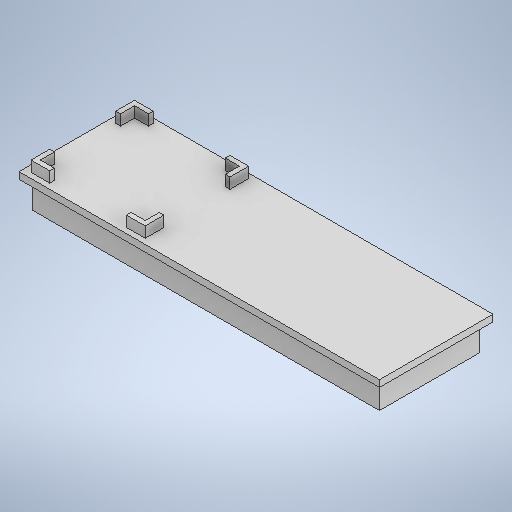
# Autodesk Inventor part: jugglingGloveCap
Saved by Autodesk Inventor 2025 (Build 290162010, 162A)
## iProperties
Created: 2024-07-10
Part Number: jugglingGloveCap
Material: Generic
Document SubType Name: Modeling
Designer: Dresden_Student
Density: 1 g/cm^3
Appearance: Default
Author: Dresden_Student
Autodesk Inventor part; units mm, degrees
ref_plane "YZ Plane" through (0, 0, 0) normal (1, 0, 0) x (0, 1, 0)
ref_plane "XZ Plane" through (0, 0, 0) normal (0, 1, 0) x (-1, 0, 0)
ref_plane "XY Plane" through (0, 0, 0) normal (0, 0, 1) x (1, 0, 0)
sketch "Sketch1" plane through (0, 0, 0) normal (0, 1, 0) x (-1, 0, 0)
  line L0 (-65, -18.75) -> (65, -18.75)
  line L1 (65, -18.75) -> (65, 18.75)
  line L2 (65, 18.75) -> (-65, 18.75)
  line L3 (-65, 18.75) -> (-65, -18.75)
  line L4 (-65, -18.75) -> (65, 18.75) construction
  line L5 (65, -18.75) -> (-65, 18.75) construction
  line L6 (61.5, 15.25) -> (-61.5, 15.25)
  line L7 (-61.5, 15.25) -> (-61.5, -15.25)
  line L8 (-61.5, -15.25) -> (61.5, -15.25)
  line L9 (61.5, -15.25) -> (61.5, 15.25)
  line L10 (61.5, 15.25) -> (-61.5, -15.25) construction
  line L11 (-61.5, 15.25) -> (61.5, -15.25) construction
  point P0 (0, 0)
  point P1 (0, 0)
  point P2 (61.5, 0)
  dimension "d0" = 37.5
  dimension "d1" = 130
  dimension "d2" = 3.5
  dimension "d3" = 3.5
  dimension "d4" = 3.5
  dimension "d5" = 3.5
  constraints: 24 end point, 5 midpoint, 4 parallel, 2 horizontal, 2 perpendicular
  measures "d0" distance of L0.end L1.end
  measures "d1" distance of L0.start L0.end
  measures "d2" distance from line of L1 point (61.5, 0)
  measures "d3" distance between parallel lines of L2 L6
  measures "d4" distance between parallel lines of L0 L8
  measures "d5" distance between parallel lines of L3 L7
extrude "Extrusion1" add sketch "Sketch1" against normal blind 2.5 contours L3 L2 L1 L0 | L9 L8 L7 L6
sketch "Sketch2" plane through (0, -2.5, 0) normal (0, -1, 0) x (1, 0, 0)
  point P0 (0, 0)
sketch "Sketch3" plane through (0, -2.5, 0) normal (0, -1, 0) x (1, 0, 0)
  line L0 (-63.875, -17.875) -> (63.875, -17.875)
  line L1 (63.875, -17.875) -> (63.875, 17.875)
  line L2 (63.875, 17.875) -> (-63.875, 17.875)
  line L3 (-63.875, 17.875) -> (-63.875, -17.875)
  line L4 (-63.875, -17.875) -> (63.875, 17.875) construction
  line L5 (63.875, -17.875) -> (-63.875, 17.875) construction
  line L6 (65, 18.75) -> (-65, 18.75) projected
  line L7 (65, -18.75) -> (65, 18.75) projected
  line L8 (-65, 18.75) -> (65, 18.75)
  line L9 (65, 18.75) -> (65, -18.75)
  line L10 (65, -18.75) -> (-65, -18.75)
  line L11 (-65, -18.75) -> (-65, 18.75)
  line L12 (-65, -18.75) -> (65, -18.75) projected
  line L13 (-65, 18.75) -> (-65, -18.75) projected
  point P0 (0, 0)
  point P1 (-65, 18.75)
  point P2 (65, -18.75)
  dimension "d8" = 0.875
  dimension "d9" = 1.125
  constraints: 20 end point, 4 collinear, 4 parallel, 2 horizontal, 2 midpoint, 2 perpendicular
  measures "d8" distance between parallel lines of L6 L2
  measures "d9" distance between parallel lines of L7 L1
extrude "Extrusion2" add sketch "Sketch3" along normal blind 7.5
sketch "Sketch4" plane through (0, 0, 0) normal (0, 1, 0) x (1, 0, 0)
  line L0 (-25.25, 17) -> (-63.25, 17)
  line L1 (-63.25, 17) -> (-63.25, -17)
  line L2 (-63.25, -17) -> (-25.25, -17)
  line L3 (-25.25, -17) -> (-25.25, 17)
  line L4 (-65, -18.75) -> (65, -18.75) projected
  line L5 (65, 18.75) -> (-65, 18.75) projected
  line L6 (-65, 18.75) -> (-65, -18.75) projected
  line L7 (-23.5, 18.75) -> (-65, 18.75)
  line L8 (-65, 18.75) -> (-65, -18.75)
  line L9 (-65, -18.75) -> (-23.5, -18.75)
  line L10 (-23.5, -18.75) -> (-23.5, 18.75)
  line L11 (-58, -17) -> (-58, -18.75)
  line L12 (-63.25, -11.75) -> (-65, -11.75)
  line L13 (-30.5, -17) -> (-30.5, -18.75)
  line L14 (-25.25, -11.75) -> (-23.5, -11.75)
  point P0 (0, 0)
  point P1 (-58, -17.875)
  point P2 (-30.5, -17.875)
  point P3 (-30.5, -18.75)
  point P4 (-65, -11.75)
  point P5 (-58, -18.75)
  dimension "d12" = 34
  dimension "d13" = 38
  dimension "d14" = 37.5
  dimension "d15" = 1.75
  dimension "d16" = 1.75
  dimension "d17" = 1.75
  dimension "d18" = 7
  dimension "d19" = 7
  dimension "d20" = 7
  dimension "d21" = 7
  constraints: 24 end point, 8 point on line, 6 perpendicular, 4 parallel, 3 collinear, 2 horizontal, 2 midpoint
  measures "d12" distance of L2.end L0.start
  measures "d13" distance of L1.end L2.end
  measures "d14" distance between parallel lines of L4 L5
  measures "d15" distance between parallel lines of L4 L2
  measures "d16" distance between parallel lines of L6 L1
  measures "d17" distance between parallel lines of L3 L10
  measures "d18" distance from line of L8 point (-58, -17.875)
  measures "d19" distance between parallel lines of L9 L12
  measures "d20" distance from line of point (-30.5, -17.875) L10
  measures "d21" distance between parallel lines of L4 L14
extrude "Extrusion3" add sketch "Sketch4" along normal blind 4 contours L14 L10 L4 L13 L2 L3 | L1 L2 L11 L4 L6 L12
mirror "Mirror1" about plane through (0, 0, 0) normal (0, 0, 1) of "Extrusion3"
move faces "Move1" translate (0, 2.5, 0) faces at (-62.0833, 4, 18.1667) (-26.4167, 4, 18.1667) (35.5, 0, 3.9167) (-26.4167, 4, -18.1667) (-62.0833, 4, -18.1667)
sketch "Sketch5" plane through (-65, -10, 18.75) normal (0, 0, 1) x (1, 0, 0)
  line L0 (0, 12.5) -> (130, 12.5)
  line L1 (130, 12.5) -> (130, 10)
  line L2 (130, 10) -> (0, 10)
  line L3 (0, 10) -> (0, 12.5)
  line L4 (41.5, 12.5) -> (130, 12.5) projected
  line L5 (130, 12.5) -> (130, 0) projected
  line L6 (0, 0) -> (0, 16.5) projected
  point P0 (65, 10)
  dimension "d27" = 2.5
  constraints: 8 end point, 3 collinear, 2 parallel, 1 horizontal, 1 perpendicular
  measures "d27" distance between parallel lines of L2 L0
sketch "Sketch6" plane through (-65, -10, -18.75) normal (-1, 0, 0) x (0, 0, 1)
  point P0 (18.75, 10)
extrude "Extrusion4" add sketch "Sketch5" along normal blind 2.5
mirror "Mirror2" about plane through (0, 0, 0) normal (0, 0, 1) of "Extrusion4"
sketch "Sketch7" plane through (-65, -10, -18.75) normal (-1, 0, 0) x (0, 0, 1)
  line L0 (-2.5, 12.5) -> (40, 12.5)
  line L1 (40, 12.5) -> (40, 10)
  line L2 (40, 10) -> (-2.5, 10)
  line L3 (-2.5, 10) -> (-2.5, 12.5)
  line L4 (40, 12.5) -> (40, 10) projected
  line L5 (-2.5, 12.5) -> (-2.5, 10) projected
  line L6 (7, 12.5) -> (30.5, 12.5) projected
  line L7 (0, 10) -> (-2.5, 10) projected
  point P0 (18.75, 10)
  constraints: 8 end point, 4 collinear, 2 parallel, 1 horizontal, 1 perpendicular
extrude "Extrusion5" add sketch "Sketch7" along normal blind 2.5
mirror "Mirror3" about plane through (0, 0, 0) normal (1, 0, 0) of "Extrusion5"
move faces "Move2" translate (0, 0, -1) faces at (-58, 3.8333, -18.1667) (-26.4167, 6.5, -18.1667) (-62.0833, 6.5, -18.1667) (-30.5, 3.8333, -17.5833) (-59.75, 3.8333, -17) (-63.8333, 3.8333, -11.75) (-60.3333, 3.8333, -18.75) (-65, 5.1667, -16.4167) (-27, 3.8333, -17) (-24.0833, 5.1667, -11.75) (-25.25, 3.8333, -13.5) (-23.5, 3.8333, -16.4167) (-25.8333, 5.1667, -18.75) (-63.25, 3.8333, -15.25)
move faces "Move3" translate (0, 0, 1) faces at (-62.0833, 6.5, 18.1667) (-63.25, 3.8333, 15.25) (-65, 3.8333, 14.0833) (-62.6667, 3.8333, 18.75) (-24.0833, 5.1667, 11.75) (-24.0833, 6.5, 15.8333) (-30.5, 3.8333, 17.5833) (-25.25, 3.8333, 13.5) (-27, 3.8333, 17) (-25.8333, 3.8333, 18.75) (-23.5, 5.1667, 16.4167) (-58, 3.8333, 18.1667) (-59.75, 3.8333, 17) (-63.8333, 3.8333, 11.75)
move faces "Move4" translate (1, 0, 0) faces at (-24.0833, 6.5, 16.8333) (-27, 3.8333, -18) (-23.5, 5.1667, 17.4167) (-24.0833, 5.1667, 12.75) (-27, 3.8333, 18) (-25.8333, 3.8333, 19.75) (-24.0833, 5.1667, -12.75) (-25.25, 3.8333, -14.5) (-23.5, 3.8333, -17.4167) (-26.4167, 6.5, -19.1667) (-25.8333, 5.1667, -19.75) (-25.25, 3.8333, 14.5) (-30.5, 3.8333, 18.5833) (-30.5, 3.8333, -18.5833)
move faces "Move5" translate (1, 0, 0) faces at (-23.0833, 6.5, 16.8333) (-22.5, 5.1667, 17.4167) (-22.5, 3.8333, -17.4167) (-23.0833, 5.1667, 12.75) (-24.25, 3.8333, 14.5) (-24.8333, 3.8333, 19.75) (-24.25, 3.8333, -14.5) (-23.0833, 5.1667, -12.75) (-25.4167, 6.5, -19.1667) (-24.8333, 5.1667, -19.75) (-26, 3.8333, -18) (-26, 3.8333, 18) (-29.5, 3.8333, -18.5833) (-29.5, 3.8333, 18.5833)
move faces "Move6" translate (-0.75, 0, 0) faces at (-23.8333, 5.1667, -19.75) (-23.8333, 3.8333, 19.75) (-28.5, 3.8333, 18.5833) (-22.0833, 5.1667, 12.75) (-25, 3.8333, 18) (-22.0833, 6.5, 16.8333) (-21.5, 5.1667, 17.4167) (-23.25, 3.8333, 14.5) (-25, 3.8333, -18) (-23.25, 3.8333, -14.5) (-28.5, 3.8333, -18.5833) (-22.0833, 5.1667, -12.75) (-21.5, 3.8333, -17.4167) (-24.4167, 6.5, -19.1667)
move faces "Move7" translate (0, 0, 0.25) faces at (-24.5833, 5.1667, -19.75) (-65, 5.1667, -17.4167) (-63.25, 5.1667, -16.25) (-59.75, 3.8333, -18) (-62.0833, 6.5, -19.1667) (-58, 3.8333, -19.1667) (-29.25, 3.8333, -18.5833) (-25.75, 3.8333, -18) (-24, 3.8333, -14.5) (-22.8333, 3.8333, -12.75) (-22.25, 3.8333, -17.4167) (-60.3333, 3.8333, -19.75) (-25.1667, 6.5, -19.1667) (-63.8333, 3.8333, -12.75)
move faces "Move8" translate (0, 0, -0.5) faces at (-65, 3.8333, 15.0833) (-63.8333, 3.8333, 12.75) (-62.6667, 3.8333, 19.75) (-29.25, 3.8333, 18.5833) (-24, 3.8333, 14.5) (-22.8333, 3.8333, 12.75) (-22.25, 5.1667, 17.4167) (-22.8333, 6.5, 16.8333) (-24.5833, 3.8333, 19.75) (-59.75, 3.8333, 18) (-25.75, 3.8333, 18) (-58, 5.1667, 19.1667) (-62.0833, 6.5, 19.1667) (-63.25, 5.1667, 16.25)
equation "\"d2\" = d3"
equation "\"d4\" = d3"
equation "\"d5\" = d3"
equation "\"d15\" = -0.5 * d12 + 0.5 * d14"
equation "\"d16\" = d15"
equation "\"d17\" = d16"
body "Solid1"
